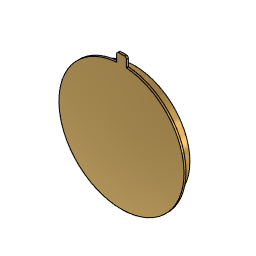
Outer Hat v8 (Autodesk Fusion 360 design; units mm, degrees)
Autodesk Fusion 360 part; units mm, degrees
sketch "Sketch1" plane through (0, 0, 0) normal (0, 1, 0) x (1, 0, 0)
  circle A0 centre (0, 0) radius 81
  circle A1 centre (0, 0) radius 85
  circle A2 centre (0, 0) radius 96
  line L0 (4.5, -110) -> (-4.5, -110)
  line L1 (-7.5, -107) -> (-7.5, -90)
  line L2 (-7.5, -90) -> (7.5, -90)
  line L3 (7.5, -90) -> (7.5, -107)
  arc A3 (4.5, -110) -> (7.5, -107) centre (4.5, -107) ccw
  arc A4 (-7.5, -107) -> (-4.5, -110) centre (-4.5, -107) ccw
  line L4 (0, 0) -> (0, -130)
  dimension "d1" = 162
  dimension "d2" = 170
  dimension "d3" = 192
  dimension "d13" = 3
  dimension "d14" = 3
  dimension "d15" = 15
  dimension "d16" = 20
  dimension "d17" = 90
  constraint coincident A0.centre A1.centre
  constraint concentric A0 A1
  constraint horizontal L0
  constraint vertical L1
  constraint horizontal L2
  constraint vertical L3
  constraint tangent L0 A3
  constraint tangent L3 A3
  constraint tangent L0 A4
  constraint tangent L1 A4
  constraint perpendicular L0 L4
  constraint symmetric L1 L3 L4
  measures "d1" diameter of A0
  measures "d2" diameter of A1
  measures "d3" diameter of A2
  measures "d13" radius of A3
  measures "d14" radius of A4
  measures "d15" distance of L1.end L2.end
  measures "d16" distance of L0 L2
  measures "d17" distance of A0.centre L2
extrude "Extrude1" add sketch "Sketch1" along normal blind 20 contours A1
extrude "Extrude2" add sketch "Sketch1" along normal blind 3 contours A0 | A2 L1 L2 L3 | A2 L1 L2 L4 | A2 L2 L3 L4
ref_plane "WorkPlane1" through (0, 5, 0) normal (0, 1, 0) x (1, 0, 0)
sketch "Sketch2" plane through (0, 5, 0) normal (0, 1, 0) x (1, 0, 0)
  line L0 (6.25, -93.8796) -> (-6.25, -93.8796)
  line L1 (-6.25, -93.8796) -> (-6.25, -70)
  line L2 (-6.25, -70) -> (6.25, -70)
  line L3 (6.25, -70) -> (6.25, -93.8796)
  line L4 (0, 0) -> (0, -104.4025)
  line L5 (3.25, -90) -> (-3.25, -90)
  line L6 (-3.25, -90) -> (-3.25, -75)
  line L7 (-3.25, -75) -> (3.25, -75)
  line L8 (3.25, -75) -> (3.25, -90)
  dimension "d18" = 12.5
  dimension "d19" = 6.5
  constraint horizontal L0
  constraint vertical L1
  constraint horizontal L2
  constraint vertical L3
  constraint coincident L4.start origin
  constraint perpendicular L0 L4
  constraint symmetric L1 L3 L4
  constraint horizontal L5
  constraint vertical L6
  constraint horizontal L7
  constraint vertical L8
  constraint symmetric L4 L6 L8
  measures "d18" distance of L1.end L2.end
  measures "d19" distance of L5.start L5.end
extrude "Extrude3" cut sketch "Sketch2" against normal blind 2
extrude "Extrude4" add sketch "Sketch1" along normal blind 3 contours A2 L0 L1 A4 L4 | A2 L0 L3 A3 L4
extrude "Extrude5" cut sketch "Sketch2" along normal blind 4 contours L4 L5 L6 L7 | L4 L5 L7 L8
fillet "Fillet1" radius 1 1 edges at (0, 3, -85)
